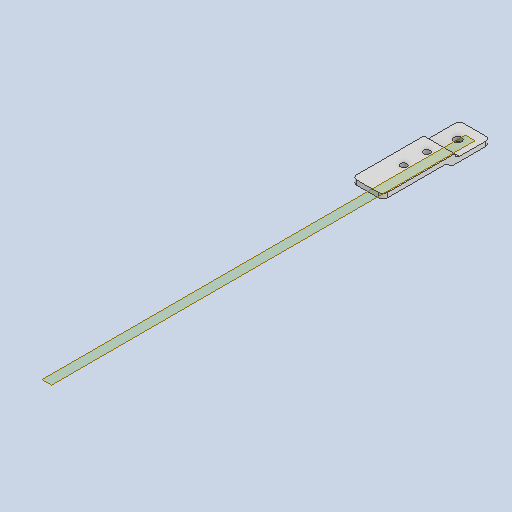
# Autodesk Inventor part: крепление шкива боковое
Saved by Autodesk Inventor 2024.2 (Build 282272000, 272)
## iProperties
Created: 2026-02-02
Part Number: крепление шкива боковое
Material: Типовые
Document SubType Name: Modeling
Designer: katya_notebook
Density: 1 g/cm^3
Appearance: По умолчанию
Author: katya_notebook
Autodesk Inventor part; units mm, degrees
ref_plane "YZ Plane" through (0, 0, 0) normal (1, 0, 0) x (0, 1, 0)
ref_plane "XZ Plane" through (0, 0, 0) normal (0, 1, 0) x (-1, 0, 0)
ref_plane "XY Plane" through (0, 0, 0) normal (0, 0, 1) x (1, 0, 0)
ref_plane "РабПлоскость1" through (-30.8415, -18.9359, 233.6055) normal (0, -1, 0) x (1, 0, 0)
sketch "Эскиз1" plane through (-30.8415, -18.9359, 233.6055) normal (0, -1, 0) x (1, 0, 0)
  line L0 (-13.3, -2.5) -> (-13.3, -252.5) projected
  line L1 (6.7, -2.5) -> (6.7, -252.5) projected
  line L2 (-13.3, -201.977) -> (6.7, -201.977)
  line L3 (6.7, -201.977) -> (6.7, -265.977)
  line L4 (0.7, -271.977) -> (-7.3, -271.977)
  line L5 (-13.3, -265.977) -> (-13.3, -201.977)
  line L6 (-6.6, -2.5) -> (-6.6, -252.5) projected
  line L7 (0, -2.5) -> (0, -252.5) projected
  circle A0 centre (-3.3, -240.5) radius 2
  circle A1 centre (-3.3, -225.5) radius 2
  line L8 (-6.2393, -252.5) -> (-3.6, -252.5) projected
  arc A2 (-13.3, -265.977) -> (-7.3, -271.977) centre (-7.3, -265.977) ccw
  arc A3 (0.7, -271.977) -> (6.7, -265.977) centre (0.7, -265.977) ccw
  circle A4 centre (-3.3, -260.5001) radius 3.3 projected
  point P0 (30.8415, -233.6055)
  point P1 (-13.3, -271.977)
  point P2 (-4.9197, -252.5)
  dimension "d0" = 70
  dimension "d1" = 15
  dimension "d2" = 4
  dimension "d3" = 4
  dimension "d4" = 3.3
  dimension "d5" = 12
  dimension "d6" = 6
  constraints: 8 end point, 4 centre point, 4 point on circle, 4 point on line, 4 tangent, 2 parallel, 1 equal radius, 1 horizontal, 1 midpoint, 1 perpendicular, 1 vertical alignment
  measures "d0" distance of point (-13.3, -271.977) L2.start
  measures "d1" distance of A1.centre A0.centre
  measures "d2" diameter of A0
  measures "d3" diameter of A1
  measures "d4" distance from line of L6 A1.centre
  measures "d5" vertical distance of point (-4.92, -252.5) A0.centre
  measures "d6" radius of A2
extrude "Выдавливание1" add sketch "Эскиз1" along normal blind 3
sketch "Эскиз2" plane through (-30.8415, -21.9359, 233.6055) normal (0, -1, 0) x (1, 0, 0)
  line L0 (-13.3, -201.977) -> (-13.3, -265.977) projected
  line L1 (-13.3, -248.5069) -> (-13.3, -271.977)
  line L2 (-13.3, -271.977) -> (6.7, -271.977)
  line L3 (6.7, -271.977) -> (6.7, -248.5069)
  line L4 (6.7, -265.977) -> (6.7, -201.977) projected
  line L5 (-13.3, -248.5069) -> (6.7, -248.5069)
  point P0 (30.8415, -233.6055)
  point P1 (0.7, -271.977)
  constraints: 8 end point, 3 point on line, 2 perpendicular, 1 collinear, 1 horizontal
extrude "Выдавливание2" cut sketch "Эскиз2" against normal blind 3
sketch "Эскиз3" plane through (-30.8415, -21.9359, 233.6055) normal (0, -1, 0) x (1, 0, 0)
  line L0 (-13.3, -201.977) -> (-13.3, -248.5069) projected
  line L1 (-13.3, -244.5069) -> (6.7, -244.5069)
  line L2 (6.7, -244.5069) -> (6.7, -271.5069)
  line L3 (6.7, -271.5069) -> (-13.3, -271.5069)
  line L4 (-13.3, -271.5069) -> (-13.3, -244.5069)
  line L5 (6.7, -248.5069) -> (6.7, -201.977) projected
  line L6 (-13.3, -248.5069) -> (6.7, -248.5069) projected
  circle A0 centre (-3.3, -260.5001) radius 2.5 projected
  point P0 (30.8415, -233.6055)
  point P1 (-13.3, -248.5069)
  dimension "d11" = 27
  dimension "d12" = 4
  constraints: 8 end point, 2 parallel, 2 point on line, 1 horizontal, 1 perpendicular
  measures "d11" distance of L3.end L1.start
  measures "d12" distance between parallel lines of L6 L1
extrude "Выдавливание3" add sketch "Эскиз3" along normal blind 3
fillet "Сопряжение1" radius 3 3 edges at (-34.1415, -21.9359, -10.9015) (-34.1415, -21.9359, -14.9015) (-34.1415, -24.9359, -10.9015)
fillet "Сопряжение2" radius 3 4 edges at (-44.1415, -23.4359, -37.9015) (-24.1415, -23.4359, -37.9015) (-44.1415, -20.4359, 31.6285) (-24.1415, -20.4359, 31.6285)
